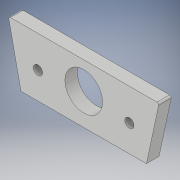
# Autodesk Inventor part: Brake_Light_Base_Plate
Saved by Autodesk Inventor 2019 (Build 230136000, 136)
## iProperties
Created: 2019-08-13
Part Number: Brake_Light_Base_Plate
Material: Generic
Document SubType Name: Modeling
Designer: steve
Density: 1 g/cm^3
Appearance: Default
topWidth: 180.000 mm
Author: steve
Autodesk Inventor part; units mm, degrees
ref_plane "YZ Plane" through (0, 0, 0) normal (1, 0, 0) x (0, 1, 0)
ref_plane "XZ Plane" through (0, 0, 0) normal (0, 1, 0) x (-1, 0, 0)
ref_plane "XY Plane" through (0, 0, 0) normal (0, 0, 1) x (1, 0, 0)
sketch "hole pattern" plane through (0, 0, 0) normal (0, 0, 1) x (1, 0, 0)
  circle A0 centre (-54.635, 0) radius 5 construction
  line L0 (-126, 0) -> (126, 0) projected
  line L1 (0, -46) -> (0, 52) projected
  circle A1 centre (0, 5.5) radius 22.5
  line L2 (-54.635, -5) -> (0, -5) construction
  circle A2 centre (54.635, 0) radius 5 construction
  line L3 (-90, 38) -> (90, 38)
  line L4 (-90, 38) -> (-75, -32)
  line L5 (-75, -32) -> (75, -32)
  line L6 (75, -32) -> (90, 38)
  circle A3 centre (-54.635, 0) radius 15 construction
  circle A4 centre (54.635, 0) radius 15 construction
  circle A5 centre (-54.635, 0) radius 5.5
  circle A6 centre (54.635, 0) radius 5.5
  point P0 (0, 0)
  dimension "d1" = 10
  dimension "d0" = 54.635
  dimension "d2" = 45
  dimension "topWidth" = 180
  dimension "d38" = 90
  dimension "d39" = 32.5
  dimension "d40" = 10.5
  dimension "d41" = 32
  dimension "d42" = 30
  dimension "d43" = 30
  dimension "d44" = 11
  dimension "d45" = 11
  dimension "d76" = 150
  constraints: 10 end point, 6 centre point, 4 coincident, 3 horizontal, 3 point on line, 1 equal length, 1 parallel, 1 perpendicular, 1 symmetric about line, 1 vertical alignment, 3 other
  measures "d0" distance of point (0, 0) point (-54.635, 0)
  measures "d2" diameter of A1
  measures "topWidth" distance of L3.start L3.end
  measures "d38" distance from line of L3.end L1
  measures "d39" distance from line of L3 A1.centre
  measures "d40" distance from line of A1.centre L2
  measures "d41" distance between parallel lines of L0 L5
  measures "d42" diameter of A3
  measures "d43" diameter of A4
  measures "d44" diameter of A5
  measures "d45" diameter of A6
  measures "d76" distance of L4.end L5.end
extrude "Extrusion1" add sketch "hole pattern" along normal blind 15 contours L4 L3 L1 A1 L0 A5 | L0 A5 A1 L1 L5 L4 | L3 L6 L0 A6 A1 L1 | L1 A1 L0 A6 L6 L5
fillet "Fillet1" radius 2 2 edges at (-90, 38, 7.5) (90, 38, 7.5)
equation "\"d38\" = 0.5 * topWidth"
body "Solid1"
